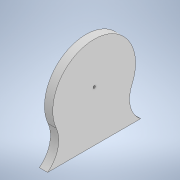
# Autodesk Inventor part: Base Hinge 2x
Saved by Autodesk Inventor 2020.2 (Build 242310000, 310)
## iProperties
Created: 2020-03-30
Part Number: Base Hinge 2x
Material: Generic
Document SubType Name: Modeling
Designer: Amaan Khalid
Density: 1 g/cm^3
Appearance: Default
Author: Amaan Khalid
Autodesk Inventor part; units mm, degrees
ref_plane "YZ Plane" through (0, 0, 0) normal (1, 0, 0) x (0, 1, 0)
ref_plane "XZ Plane" through (0, 0, 0) normal (0, 1, 0) x (-1, 0, 0)
ref_plane "XY Plane" through (0, 0, 0) normal (0, 0, 1) x (1, 0, 0)
sketch "Sketch1" plane through (0, 0, 0) normal (1, 0, 0) x (0, 1, 0)
  arc A0 (-10.9904, -24.3236) -> (-10.9904, 33.6895) centre (1.9201, 4.683) ccw
  arc A1 (-36.9675, 40.4029) -> (-10.9904, 33.6895) centre (-19.7566, 53.3848) ccw
  arc A2 (-10.9904, -24.3236) -> (-36.9675, -31.0369) centre (-19.7566, -44.0189) ccw
  line L0 (-36.9675, 40.4029) -> (-36.9675, -31.0369)
  circle A3 centre (1.9201, 4.683) radius 0.9144
  dimension "d1" = 1.8288
  constraints: 6 point on circle, 4 centre point, 2 end point, 1 coincident, 1 tangent, 1 vertical
  measures "d1" diameter of A3
extrude "Extrusion1" add sketch "Sketch1" along normal blind 6.35
body "Solid1"
